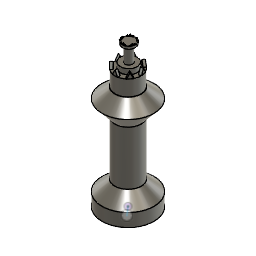
chess- king (Autodesk Fusion 360 design; units mm, degrees)
part number: 2026-07-02-15-21-05-411
Autodesk Fusion 360 part; units mm, degrees
sketch "Sketch1" plane through (0, 0, 0) normal (0, 0, 1) x (1, 0, 0)
sketch "Sketch2" plane through (0, 0, 0) normal (0, 0, 1) x (1, 0, 0)
  line L0 (0, 0) -> (0, 50.8)
  line L1 (0, 0) -> (12.7, 0)
  line L2 (12.7, 0) -> (12.7, 6.385)
  line L3 (12.7, 6.385) -> (12.7, 0)
  line L4 (0, 50.8) -> (6.472, 50.8)
  line L5 (6.472, 50.8) -> (12.7, 45.72)
  line L6 (6.472, 11.8034) -> (12.7, 6.385)
  line L7 (6.472, 11.8034) -> (6.472, 38.1)
  line L8 (6.472, 38.1) -> (12.7, 45.72)
  constraint coincident L0.start L1.start
  constraint vertical L0
  constraint perpendicular L0 L1
  constraint perpendicular L1 L2
  constraint perpendicular L0 L4
  constraint parallel L3 L7
revolve "Revolve1" add sketch "Sketch2" angle 360 about axis through (0, 0, 0) along (0, 1, 0) makes body 1
sketch "Sketch3" plane through (0, 0, 0) normal (0, 0, 1) x (1, 0, 0)
sketch "Sketch4" plane through (0, 0, 0) normal (0, 1, 0) x (1, 0, 0)
  circle A0 centre (38.1, 0) radius 6.35
  dimension "d3" = 12.7
  measures "d3" diameter of A0
extrude "Extrude1" add sketch "Sketch4" along normal blind 7.62 separate body makes body 2
sketch "Sketch5" plane through (0, 7.62, 0) normal (0, 1, 0) x (-1, 0, 0)
  circle A0 centre (-38.1, 0) radius 6.35
  circle A1 centre (-38.1, 0) radius 3.81
  dimension "d6" = 7.62
  constraint concentric A0 A1
  measures "d6" diameter of A1
extrude "Extrude2" cut sketch "Sketch5" against normal blind 2540 contours A1 bodies 2
ref_plane "WorkPlane1" through (38.1, 4.0537, 6.35) normal (0, 0, 1) x (-1, 0, 0)
sketch "Sketch6" plane through (0, 0, 6.35) normal (0, 0, 1) x (1, 0, 0)
  line L0 (44.45, 7.62) -> (31.75, 7.62)
  line L1 (44.45, 0) -> (31.75, 0)
  line L2 (36.83, 7.62) -> (38.1, 10.16)
  line L3 (38.1, 10.16) -> (39.37, 7.62)
  line L4 (39.37, 7.62) -> (36.83, 7.62)
  constraint coincident L0 L2.start
  constraint coincident L0 L3.end
extrude "Extrude3" add sketch "Sketch6" against normal blind 1.27 bodies 2
pattern_circular "C-Pattern1" count 7 over 360 about axis through (38.1, 7.62, 0) along (0, 1, 0) of "Extrude3"
move_body "Move1" bodies 2 to x (1, 0, 0) y (0, 1, 0) z (0, 0, 1) at (-38.1, 50.8, 1.27)
move_body "Move2" bodies 2 to x (1, 0, 0) y (0, 1, 0) z (0, 0, 1) at (0, 0, -1.27)
sketch "Sketch7" plane through (0, 0, 0) normal (0, 1, 0) x (1, 0, 0)
move_body "Move3" bodies 2 to x (1, 0, 0) y (0, 1, 0) z (0, 0, 1) at (38.1, 0, 0)
sketch "Sketch8" plane through (0, 50.8, 0) normal (0, 1, 0) x (-1, 0, 0)
  circle A0 centre (0, 0) radius 6.472
  circle A1 centre (0, 0) radius 5.08
  dimension "d14" = 10.16
  constraint concentric A0 A1
  measures "d14" diameter of A1
extrude "Extrude4" cut sketch "Sketch8" against normal blind 48.26 contours A1 bodies 1
move_body "Move4" bodies 2 to x (1, 0, 0) y (0, 1, 0) z (0, 0, 1) at (-38.1, 0, 0)
sketch "Sketch9" plane through (0, 0, 0) normal (0, 1, 0) x (1, 0, 0)
sketch "Sketch10" plane through (0, 0, 0) normal (0, 0, 1) x (1, 0, 0)
sketch "Sketch11" plane through (0, 0, 0) normal (0, 1, 0) x (1, 0, 0)
  circle A0 centre (50.8, 0) radius 4.064
  dimension "d18" = 8.128
  measures "d18" diameter of A0
extrude "Extrude5" add sketch "Sketch11" along normal blind 2.54 separate body makes body 3
sketch "Sketch13" plane through (0, 0, 0) normal (0, 0, 1) x (1, 0, 0)
  line L0 (25.4, -25.4) -> (27.432, -25.4)
  line L1 (27.432, -25.4) -> (27.432, 5.08)
  line L2 (25.4, -25.4) -> (25.4, 10.16)
  line L3 (25.4, 10.16) -> (27.432, 5.08)
  dimension "d23" = 2.032
  constraint horizontal L0
  constraint perpendicular L0 L1
  constraint perpendicular L0 L2
  measures "d23" distance of L0.start L0.end
sketch "Sketch15" plane through (0, 0, 0) normal (0, 0, 1) x (1, 0, 0)
  line L0 (-19.05, 0) -> (-24.13, 0)
  line L1 (-24.13, 0) -> (-24.13, 20.32)
  line L2 (-19.05, 0) -> (-19.05, 25.4)
  line L3 (-24.13, 20.32) -> (-19.05, 25.4)
  dimension "d30" = 5.08
  dimension "d31" = 20.32
  dimension "d32" = 25.4
  constraint horizontal L0
  constraint perpendicular L0 L1
  constraint perpendicular L0 L2
  measures "d30" distance of L0.start L0.end
  measures "d31" distance of L0.end L1.end
  measures "d32" distance of L0.start L2.end
extrude "Extrude8" add sketch "Sketch15" along normal blind 2.54 separate body makes body 4
move_body "Move7" bodies 4 to x (1, 0, 0) y (0, 1, 0) z (0, 0, 1) at (71.12, 0, -3.81)
move_body "Move8" bodies 4 to x (1, 0, 0) y (0, 1, 0) z (0, 0, 1) at (1.778, 2.54, 2.54)
move_body "Move9" bodies 4 to x (1, 0, 0) y (0, 1, 0) z (0, 0, 1) at (-0.254, 0, 0)
sketch "Sketch16" plane through (0, 0, 0) normal (0, -1, 0) x (1, 0, 0)
  circle A0 centre (50.8, 0) radius 4.064
  circle A1 centre (50.8, 0) radius 1.905
  dimension "d35" = 3.81
  constraint concentric A0 A1
  measures "d35" diameter of A1
extrude "Extrude9" add sketch "Sketch16" along normal blind 7.62 contours A1 bodies 3
combine "Combine1" operation add target body 3 tool bodies 4
move_body "Move10" bodies 3 to x (-1, 0, 0) y (0, -1, 0) z (0, 0, 1) at (93.472, -15.24, 0)
move_body "Move11" bodies 3 to x (1, 0, 0) y (0, 1, 0) z (0, 0, 1) at (-43.18, 86.36, 0)
move_body "Move12" bodies 3 to x (1, 0, 0) y (0, 1, 0) z (0, 0, 1) at (0.508, 0, 0)
move_body "Move13" bodies 3 to x (1, 0, 0) y (0, 1, 0) z (0, 0, 1) at (0, -10.16, 0)
sketch "Sketch17" plane through (0, 0, 0) normal (0, 1, 0) x (1, 0, 0)
  circle A0 centre (38.1, 0) radius 3.175
  dimension "d38" = 6.35
  measures "d38" diameter of A0
extrude "Extrude10" add sketch "Sketch17" along normal blind 1.27 separate body makes body 5
ref_plane "WorkPlane2" through (38.1, 0.8968, 3.175) normal (0, 0, 1) x (-1, 0, 0)
sketch "Sketch18" plane through (0, 0, 3.175) normal (0, 0, 1) x (1, 0, 0)
  line L0 (41.275, 1.27) -> (34.925, 1.27)
  line L1 (41.275, 0) -> (34.925, 0)
  line L2 (37.465, 1.27) -> (38.1, 1.905)
  line L3 (38.1, 1.905) -> (38.735, 1.27)
  line L4 (38.735, 1.27) -> (39.0604, 1.6512)
  line L5 (39.0604, 1.6512) -> (39.37, 1.27)
  line L6 (37.465, 1.27) -> (37.1554, 1.6512)
  line L7 (37.1554, 1.6512) -> (36.83, 1.27)
  constraint coincident L0 L2.start
  constraint coincident L0 L3.end
  constraint perpendicular L2 L3
  constraint coincident L0 L5.end
  constraint parallel L5 L6
  constraint coincident L0 L7.end
extrude "Extrude11" add sketch "Sketch18" against normal blind 0.508 separate body makes body 6 at (38.3117, 1.27, 3.0057)
pattern_circular "C-Pattern2" count 5 over 360 about axis through (38.1, 1.27, 0) along (0, 1, 0) of "Extrude11" makes body 7 makes body 8 makes body 9 makes body 10
sketch "Sketch19" plane through (0, 0, 0) normal (0, 0, 1) x (1, 0, 0)
  arc A0 (31.75, 12.7) -> (34.2176, 10.5116) centre (31.5424, 9.9805) ccw
  arc A1 (34.2176, 10.5116) -> (39.8208, 9.2268) centre (36.5591, 7.8629) ccw
  arc A2 (31.75, 12.7) -> (34.2176, 10.5116) centre (31.9157, 10.4015) ccw
  arc A3 (34.2176, 10.5116) -> (39.8208, 9.2268) centre (36.6702, 8.3472) ccw
  arc A4 (29.7327, 4.7656) -> (34.2176, 10.5116) centre (29.4954, 9.5741) ccw
  arc A5 (29.7327, 5.6579) -> (34.2176, 10.5116) centre (30.2098, 9.7159) ccw
  line L0 (29.7327, 4.7656) -> (29.7327, 5.6579)
  arc A6 (29.7327, 5.6579) -> (26.67, 2.54) centre (28.8016, 3.5093) ccw
  arc A7 (29.7327, 4.7656) -> (27.94, 2.54) centre (29.1089, 3.4333) ccw
  line L1 (26.67, 2.54) -> (27.94, 2.54)
  arc A8 (28.194, 11.938) -> (30.48, 12.954) centre (28.8561, 13.5279) ccw
  arc A9 (28.194, 11.938) -> (30.48, 12.954) centre (28.0062, 15.4403) ccw
  constraint tangent A0 A4
  constraint tangent A0 A5
  constraint vertical L0
  constraint horizontal L1
  constraint tangent A0 A8
combine "Combine2" operation add target body 7 tool bodies 9 5 6 10 8
move_body "Move16" bodies 7 to x (1, 0, 0) y (0, 1, 0) z (0, 0, 1) at (-40.3419, 68.834, -13.1079)
move_body "Move17" bodies 7 to x (1, 0, 0) y (0, 1, 0) z (0, 0, 1) at (2.54, 0, 11.43)
sketch "Sketch20" plane through (0, 0, 0) normal (0, 1, 0) x (1, 0, 0)
  circle A0 centre (38.1, 0) radius 0.635
  dimension "d48" = 1.27
  measures "d48" diameter of A0
move_body "Move23" bodies 7 to x (1, 0, 0) y (0, 1, 0) z (0, 0, 1) at (60.96, -43.18, 0)
move_body "Move24" bodies 7 to x (1, 0, 0) y (0, 1, 0) z (0, 0, 1) at (0, -25.4, 0)
move_body "Move28" bodies 3 to x (-1, 0, 0) y (0, -1, 0) z (0, 0, 1) at (75.692, 68.58, 0)
combine "Combine3" operation add target body 2 tool bodies 1
move_body "Move31" bodies 3 to x (-0.965926, 0, 0.258819) y (0, -1, 0) z (0.258819, 0, 0.965926) at (75.624, 68.58, -0.9274)
move_body "Move32" bodies 3 to x (1, 0, 0) y (0, 1, 0) z (0, 0, 1) at (-2.54, 0, -17.78)
move_body "Move34" bodies 7 to x (1, 0, 0) y (0, 1, 0) z (0, 0, 1) at (-38.1, 0, 0)
sketch "Sketch21" plane through (0, 0, 0) normal (0, 0, 1) x (1, 0, 0)
  line L0 (0, 0) -> (-0.5537, -4.1088)
  constraint coincident L0.start origin
move_body "Move35" bodies 3 to x (1, 0, 0) y (0, 1, 0) z (0, 0, 1) at (0, 0, -1.27)
move_body "Move36" bodies 7 to x (1, 0, 0) y (0, 1, 0) z (0, 0, 1) at (-22.86, 68.58, 0)
move_body "Move37" bodies 7 to x (1, 0, 0) y (0, 1, 0) z (0, 0, 1) at (-0.254, -0.254, 0)
move_body "Move38" bodies 7 to x (1, 0, 0) y (0, 1, 0) z (0, 0, 1) at (0, 0, 1.27)
move_body "Move39" bodies 3 7 to x (1, 0, 0) y (0, 1, 0) z (0, 0, 1) at (0, 38.1, 0)
move_body "Move40" bodies 7 3 to x (1, 0, 0) y (0, 1, 0) z (0, 0, 1) at (0, -38.1, 0)
sketch "Sketch14" plane through (0, 0, 0) normal (0, -1, 0) x (1, 0, 0)
  circle A0 centre (50.8, 0) radius 4.064
  circle A1 centre (50.8, 0) radius 1.905
  dimension "d27" = 3.81
  constraint concentric A0 A1
  measures "d27" diameter of A1
extrude "Extrude7" [suppressed]
named bodies: "main", "sword", "cap"
